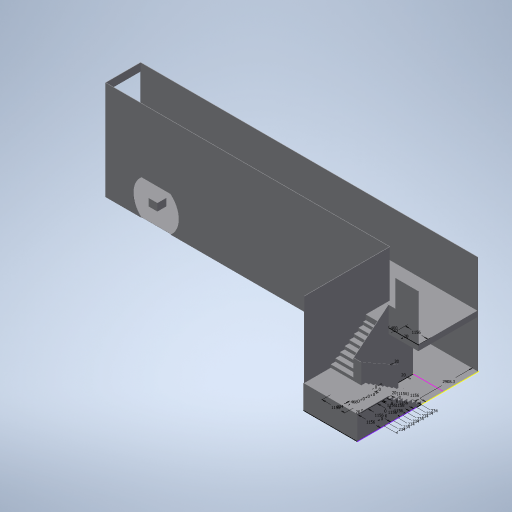
# Autodesk Inventor part: ATF_Corridors_Drawing
Saved by Autodesk Inventor 2023.1 (Build 271208000, 208)
## iProperties
Created: 2014-01-16
Part Number: ATF_Corridors_Drawing
Material: Generic
Document SubType Name: Modeling
Designer: mcgratta
Density: 1 g/cm^3
Appearance: Default
Author: mcgratta
Autodesk Inventor part; units mm, degrees
ref_plane "YZ Plane" through (0, 0, 0) normal (1, 0, 0) x (0, 1, 0)
ref_plane "XZ Plane" through (0, 0, 0) normal (0, 1, 0) x (-1, 0, 0)
sketch "Sketch1" plane through (0, 0, 0) normal (0, 1, 0) x (-1, 0, 0)
  line L0 (0, 0) -> (14380, 0)
  line L1 (14380, 0) -> (14380, -1790)
  line L2 (14380, -1790) -> (0, -1790)
  line L3 (0, -1790) -> (0, 0)
  line L4 (0, -1790) -> (-2720, -1790)
  line L5 (-2720, -1790) -> (-2720, 4350)
  line L6 (-2720, 4350) -> (0, 4350)
  line L7 (0, 4350) -> (0, -1790)
  dimension "d0" = 1790
  dimension "d2" = 14380
  dimension "d3" = 2720
  dimension "d4" = 6140
  constraints: 16 end point, 4 parallel, 2 horizontal, 2 perpendicular
  measures "d0" distance between parallel lines of L0 L2
  measures "d2" distance between parallel lines of L3 L1
  measures "d3" distance between parallel lines of L5 L7
  measures "d4" distance between parallel lines of L6 L4
extrude "Extrusion1" add sketch "Sketch1" along normal blind 10
sketch "Sketch2" plane through (0, 10, 0) normal (0, 1, 0) x (1, 0, 0)
  line L0 (2720, -4350) -> (2720, 1790) projected
  line L1 (0, -4350) -> (2720, -4350)
  line L2 (2720, -4350) -> (2720, -4330)
  line L3 (2720, -4330) -> (0, -4330)
  line L4 (0, -4330) -> (0, -4350)
  dimension "d7" = 20
  constraints: 8 end point, 2 parallel, 1 horizontal, 1 perpendicular, 1 point on line
  measures "d7" distance between parallel lines of L3 L1
extrude "Extrusion2" [suppressed]
sketch "Sketch3" plane through (0, 10, 0) normal (0, 1, 0) x (1, 0, 0)
  line L0 (2720, 1790) -> (-14380, 1790) projected
  line L1 (2720, -4330) -> (2700, -4330)
  line L2 (2700, -4330) -> (2700, 1790)
  line L3 (2700, 1790) -> (2720, 1790)
  line L4 (2720, 1790) -> (2720, -4330)
  dimension "d11" = 20
  constraints: 8 end point, 2 parallel, 1 horizontal, 1 perpendicular, 1 point on line
  measures "d11" distance between parallel lines of L4 L2
sketch "Sketch4" plane through (0, 10, 0) normal (0, 1, 0) x (1, 0, 0)
  line L0 (-14380, 1790) -> (-14380, 0) projected
  line L1 (2700, 1790) -> (-14380, 1790)
  line L2 (-14380, 1790) -> (-14380, 1770)
  line L3 (-14380, 1770) -> (2700, 1770)
  line L4 (2700, 1770) -> (2700, 1790)
  dimension "d15" = 20
  constraints: 8 end point, 2 parallel, 1 horizontal, 1 perpendicular, 1 point on line
  measures "d15" distance between parallel lines of L3 L1
extrude "Extrusion4" add sketch "Sketch4" along normal blind 5000
sketch "Sketch5" plane through (0, 10, 0) normal (0, 1, 0) x (1, 0, 0)
  line L0 (-14380, 0) -> (0, 0) projected
  line L1 (-14380, 1770) -> (-14360, 1770)
  line L2 (-14360, 1770) -> (-14360, 0)
  line L3 (-14360, 0) -> (-14380, 0)
  line L4 (-14380, 0) -> (-14380, 1770)
  dimension "d19" = 20
  constraints: 8 end point, 2 parallel, 1 horizontal, 1 perpendicular, 1 point on line
  measures "d19" distance between parallel lines of L2 L4
extrude "Extrusion5" add sketch "Sketch5" along normal blind 5000
sketch "Sketch6" plane through (0, 10, 0) normal (0, 1, 0) x (1, 0, 0)
  line L0 (-14360, 0) -> (0, 0)
  line L1 (0, 0) -> (0, 20)
  line L2 (0, 20) -> (-14360, 20)
  line L3 (-14360, 20) -> (-14360, 0)
  dimension "d23" = 20
  constraints: 8 end point, 2 parallel, 1 horizontal, 1 perpendicular
  measures "d23" distance between parallel lines of L0 L2
extrude "Extrusion6" add sketch "Sketch6" along normal blind 5000
sketch "Sketch7" plane through (0, 10, 0) normal (0, 1, 0) x (1, 0, 0)
  line L0 (0, 0) -> (0, -4350) projected
  line L1 (0, -4330) -> (2720, -4330) projected
  line L2 (0, 0) -> (20, 0)
  line L3 (20, 0) -> (20, -4330)
  line L4 (20, -4330) -> (0, -4330)
  line L5 (0, -4330) -> (0, 0)
  point P0 (2700, -4330)
  dimension "d27" = 20
  constraints: 8 end point, 2 parallel, 1 horizontal, 1 perpendicular, 1 point on line
  measures "d27" distance between parallel lines of L3 L5
extrude "Extrusion7" add sketch "Sketch7" along normal blind 5000
ref_plane "Work Plane1" through (2690, 10, 4330) normal (-1, 0, 0) x (0, 0, 1)
sketch "Sketch12" plane through (0, 10, 0) normal (0, 1, 0) x (1, 0, 0)
  line L0 (-14360, 1770) -> (-14360, 20) projected
  line L1 (-14360, 20) -> (0, 20) projected
  line L2 (-12860, 1120) -> (-12410, 1120)
  line L3 (-12410, 1120) -> (-12410, 670)
  line L4 (-12410, 670) -> (-12860, 670)
  line L5 (-12860, 670) -> (-12860, 1120)
  dimension "d115" = 1500
  dimension "d116" = 450
  dimension "d117" = 450
  dimension "d118" = 650
  constraints: 8 end point, 2 parallel, 1 horizontal, 1 perpendicular
  measures "d115" distance between parallel lines of L5 L0
  measures "d116" distance between parallel lines of L4 L2
  measures "d117" distance between parallel lines of L3 L5
  measures "d118" distance between parallel lines of L1 L4
extrude "Extrusion12" add sketch "Sketch12" along normal blind 370
sketch "Sketch13" plane through (-14360, 10, -1770) normal (1, 0, 0) x (0, 0, -1)
  line L0 (-1750, 5000) -> (-1750, 0) projected
  line L1 (0, 0) -> (-1750, 0) projected
  line L2 (0, 5000) -> (0, 0) projected
  line L3 (-1750, 5000) -> (0, 5000) projected
  line L4 (-1750, 2650) -> (0, 2650)
  line L5 (0, 2650) -> (0, 2370)
  line L6 (0, 2370) -> (-1750, 2370)
  line L7 (-1750, 2370) -> (-1750, 2650)
  point P0 (-1770, -10)
  dimension "d121" = 2370
  dimension "d122" = 2350
  constraints: 8 end point, 2 parallel, 2 point on line, 1 horizontal, 1 perpendicular
  measures "d121" distance between parallel lines of L1 L6
  measures "d122" distance between parallel lines of L4 L3
extrude "Extrusion13" add sketch "Sketch13" along normal blind 17040 contours L4 L2 L6 L0
sketch "Sketch14" plane through (0, 2380, -20) normal (0, 0, 1) x (1, 0, 0)
  line L0 (0, 0) -> (0, 280) projected
  line L1 (0, 0) -> (2680, 0) projected
  line L2 (0, 280) -> (2680, 280)
  line L3 (2680, 280) -> (2680, 0)
  line L4 (2680, 0) -> (0, 0)
  line L5 (0, 0) -> (0, 280)
  point P0 (0, -2380)
  constraints: 8 end point, 2 parallel, 1 horizontal, 1 perpendicular
extrude "Extrusion14" add sketch "Sketch14" along normal blind 1239
sketch "Sketch16" plane through (-14360, 2660, -20) normal (0, 1, 0) x (1, 0, 0)
  line L0 (17040, -1239) -> (15884, -1239)
  line L1 (15884, -1239) -> (15884, -1219)
  line L2 (15884, -1219) -> (17040, -1219)
  line L3 (17040, -1219) -> (17040, -1239)
  line L4 (15884, -1239) -> (15484, -1239)
  line L5 (15484, -1239) -> (15484, -1219)
  line L6 (15484, -1219) -> (15884, -1219)
  line L7 (15884, -1219) -> (15884, -1239)
  dimension "d168" = 20
  dimension "d170" = 1156
  dimension "d258" = 20
  dimension "d259" = 400
  constraints: 16 end point, 4 parallel, 2 horizontal, 2 perpendicular
  measures "d168" distance between parallel lines of L2 L0
  measures "d170" distance of L2.end L1.end
  measures "d258" distance between parallel lines of L6 L4
  measures "d259" distance of L5.end L6.end
extrude "Extrusion17" add sketch "Sketch16" along normal blind 2347 contours L0 L1 L2 L3
sketch "Sketch17" plane through (-14380, 0, -1790) normal (-1, 0, 0) x (0, 0, 1)
  line L0 (0, 5010) -> (1790, 5010) projected
  line L1 (20, 2663) -> (1770, 2663)
  line L2 (1770, 2663) -> (1770, 4619)
  line L3 (1770, 4619) -> (20, 4619)
  line L4 (20, 4619) -> (20, 2663)
  line L5 (0, 0) -> (0, 5010) projected
  dimension "d179" = 20
  dimension "d180" = 1750
  dimension "d181" = 391
  dimension "d182" = 1956
  constraints: 8 end point, 2 parallel, 1 horizontal, 1 perpendicular
  measures "d179" distance between parallel lines of L5 L4
  measures "d180" distance between parallel lines of L2 L4
  measures "d181" distance between parallel lines of L3 L0
  measures "d182" distance between parallel lines of L1 L3
extrude "Extrusion18" cut sketch "Sketch17" along normal mid plane 50
sketch "Sketch18" plane through (-14380, 0, 0) normal (0, 0, 1) x (1, 0, 0)
  line L0 (0, 0) -> (14380, 0) projected
  arc A0 (3305.7392, 0) -> (1827.2099, 0) centre (2566.4746, 886.2602) ccw
  constraints: 2 point on circle, 2 point on line, 1 centre point
extrude "Extrusion19" cut sketch "Sketch18" along normal mid plane 50
sketch "Sketch19" plane through (0, 10, 0) normal (0, 1, 0) x (1, 0, 0)
  line L0 (2720, -4350) -> (2720, 1790) projected
  line L1 (2720, -1118.3) -> (1564, -1118.3)
  line L2 (1564, -1118.3) -> (1564, -1352.3)
  line L3 (1564, -1352.3) -> (2720, -1352.3)
  line L4 (2720, -1352.3) -> (2720, -1118.3)
  line L5 (2700, 1790) -> (-14380, 1790) projected
  line L6 (2720, -1352.3) -> (1564, -1352.3)
  line L7 (1564, -1352.3) -> (1564, -1586.3)
  line L8 (1564, -1586.3) -> (2720, -1586.3)
  line L9 (2720, -1586.3) -> (2720, -1352.3)
  line L10 (2720, -1586.3) -> (1564, -1586.3)
  line L11 (1564, -1586.3) -> (1564, -1820.3)
  line L12 (1564, -1820.3) -> (2720, -1820.3)
  line L13 (2720, -1820.3) -> (2720, -1586.3)
  line L14 (2720, -1820.3) -> (1564, -1820.3)
  line L15 (1564, -1820.3) -> (1564, -2054.3)
  line L16 (1564, -2054.3) -> (2720, -2054.3)
  line L17 (2720, -2054.3) -> (2720, -1820.3)
  line L18 (2720, -2054.3) -> (1564, -2054.3)
  line L19 (1564, -2054.3) -> (1564, -2288.3)
  line L20 (1564, -2288.3) -> (2720, -2288.3)
  line L21 (2720, -2288.3) -> (2720, -2054.3)
  line L22 (2720, -2288.3) -> (1564, -2288.3)
  line L23 (1564, -2288.3) -> (1564, -2522.3)
  line L24 (1564, -2522.3) -> (2720, -2522.3)
  line L25 (2720, -2522.3) -> (2720, -2288.3)
  line L26 (2720, -2522.3) -> (1564, -2522.3)
  line L27 (1564, -2522.3) -> (1564, -2756.3)
  line L28 (1564, -2756.3) -> (2720, -2756.3)
  line L29 (2720, -2756.3) -> (2720, -2522.3)
  line L30 (2720, -2756.3) -> (1564, -2756.3)
  line L31 (1564, -2756.3) -> (1564, -2990.3)
  line L32 (1564, -2990.3) -> (2720, -2990.3)
  line L33 (2720, -2990.3) -> (2720, -2756.3)
  line L34 (0, 0) -> (0, -4350) projected
  line L35 (2720, -2990.3) -> (0, -2990.3)
  line L36 (0, -2990.3) -> (0, -4350)
  line L37 (0, -4350) -> (2720, -4350)
  line L38 (2720, -4350) -> (2720, -2990.3)
  line L39 (0, -2990.3) -> (1156, -2990.3)
  line L40 (1156, -2990.3) -> (1156, -2756.3)
  line L41 (1156, -2756.3) -> (0, -2756.3)
  line L42 (0, -2756.3) -> (0, -2990.3)
  line L43 (0, -2756.3) -> (1156, -2756.3)
  line L44 (1156, -2756.3) -> (1156, -2522.3)
  line L45 (1156, -2522.3) -> (0, -2522.3)
  line L46 (0, -2522.3) -> (0, -2756.3)
  line L47 (0, -2522.3) -> (1156, -2522.3)
  line L48 (1156, -2522.3) -> (1156, -2288.3)
  line L49 (1156, -2288.3) -> (0, -2288.3)
  line L50 (0, -2288.3) -> (0, -2522.3)
  line L51 (0, -2288.3) -> (1156, -2288.3)
  line L52 (1156, -2288.3) -> (1156, -2054.3)
  line L53 (1156, -2054.3) -> (0, -2054.3)
  line L54 (0, -2054.3) -> (0, -2288.3)
  line L55 (0, -2054.3) -> (1156, -2054.3)
  line L56 (1156, -2054.3) -> (1156, -1820.3)
  line L57 (1156, -1820.3) -> (0, -1820.3)
  line L58 (0, -1820.3) -> (0, -2054.3)
  line L59 (0, -1820.3) -> (1156, -1820.3)
  line L60 (1156, -1820.3) -> (1156, -1586.3)
  line L61 (1156, -1586.3) -> (0, -1586.3)
  line L62 (0, -1586.3) -> (0, -1820.3)
  line L63 (0, -1586.3) -> (1156, -1586.3)
  line L64 (1156, -1586.3) -> (1156, -1352.3)
  line L65 (1156, -1352.3) -> (0, -1352.3)
  line L66 (0, -1352.3) -> (0, -1586.3)
  line L67 (0, -1352.3) -> (1156, -1352.3)
  line L68 (1156, -1352.3) -> (1156, -1118.3)
  line L69 (1156, -1118.3) -> (0, -1118.3)
  line L70 (0, -1118.3) -> (0, -1352.3)
  line L71 (-11062.4346, 20) -> (0, 20) projected
  line L72 (0, 20) -> (1156, 20)
  line L73 (1156, 20) -> (1156, 0)
  line L74 (1156, 0) -> (0, 0)
  line L75 (0, 0) -> (0, 20)
  line L76 (0, 20) -> (2680, 20) projected
  line L77 (1156, -2990.3) -> (1176, -2990.3)
  line L78 (1176, -2990.3) -> (1176, 20)
  line L79 (1176, 20) -> (1156, 20)
  line L80 (1156, 20) -> (1156, -2990.3)
  line L81 (1564, -2990.3) -> (1544, -2990.3)
  line L82 (1544, -2990.3) -> (1544, -1118.3)
  line L83 (1544, -1118.3) -> (1564, -1118.3)
  line L84 (1564, -1118.3) -> (1564, -2990.3)
  line L85 (1544, -2990.3) -> (1176, -2990.3)
  line L86 (1176, -2990.3) -> (1176, -2970.3)
  line L87 (1176, -2970.3) -> (1544, -2970.3)
  line L88 (1544, -2970.3) -> (1544, -2990.3)
  point P0 (0, -2756.3)
  point P1 (0, -2522.3)
  point P2 (0, -2288.3)
  point P3 (0, -2054.3)
  point P4 (0, -1820.3)
  point P5 (0, -1586.3)
  point P6 (0, -1352.3)
  point P7 (0, -1118.3)
  dimension "d183" = 2908.3
  dimension "d184" = 234
  dimension "d185" = 1156
  dimension "d186" = 234
  dimension "d187" = 234
  dimension "d188" = 234
  dimension "d189" = 234
  dimension "d190" = 234
  dimension "d191" = 234
  dimension "d192" = 234
  dimension "d193" = 1156
  dimension "d194" = 0
  dimension "d195" = 0
  dimension "d196" = 0
  dimension "d197" = 0
  dimension "d198" = 0
  dimension "d199" = 0
  dimension "d200" = 0
  dimension "d201" = 1156
  dimension "d202" = 1156
  dimension "d203" = 1156
  dimension "d204" = 1156
  dimension "d205" = 1156
  dimension "d206" = 1156
  dimension "d207" = 1156
  dimension "d208" = 234
  dimension "d209" = 1156
  dimension "d210" = 0
  dimension "d211" = 0
  dimension "d212" = 0
  dimension "d213" = 0
  dimension "d214" = 0
  dimension "d215" = 0
  dimension "d216" = 468
  dimension "d251" = 20
  dimension "d252" = 20
  dimension "d253" = 20
  dimension "d268" = 20
  constraints: 168 end point, 42 parallel, 21 horizontal, 21 perpendicular, 3 point on line
  measures "d183" distance between parallel lines of L5 L1
  measures "d184" distance between parallel lines of L1 L3
  measures "d185" distance between parallel lines of L0 L2
  measures "d186" distance between parallel lines of L6 L8
  measures "d187" distance between parallel lines of L10 L12
  measures "d188" distance between parallel lines of L14 L16
  measures "d189" distance between parallel lines of L18 L20
  measures "d190" distance between parallel lines of L22 L24
  measures "d191" distance between parallel lines of L26 L28
  measures "d192" distance between parallel lines of L30 L32
  measures "d193" distance of L1.start L1.end
  measures "d194" distance between parallel lines of L6 L3
  measures "d195" distance between parallel lines of L10 L8
  measures "d196" distance between parallel lines of L12 L14
  measures "d197" distance between parallel lines of L22 L20
  measures "d198" distance between parallel lines of L16 L18
  measures "d199" distance between parallel lines of L24 L26
  measures "d200" distance between parallel lines of L28 L30
  measures "d201" distance between parallel lines of L0 L7
  measures "d202" distance between parallel lines of L0 L11
  measures "d203" distance between parallel lines of L0 L15
  measures "d204" distance between parallel lines of L0 L19
  measures "d205" distance between parallel lines of L0 L23
  measures "d206" distance between parallel lines of L0 L27
  measures "d207" distance between parallel lines of L0 L31
  measures "d208" distance between parallel lines of L41 L35
  measures "d209" distance between parallel lines of L40 L34
  measures "d210" distance between parallel lines of L47 L45
  measures "d211" distance between parallel lines of L51 L49
  measures "d212" distance between parallel lines of L55 L53
  measures "d213" distance between parallel lines of L59 L57
  measures "d214" distance between parallel lines of L61 L63
  measures "d215" distance between parallel lines of L65 L67
  measures "d216" distance between parallel lines of L47 L35
  measures "d251" distance between parallel lines of L72 L74
  measures "d252" distance between parallel lines of L78 L80
  measures "d253" distance between parallel lines of L2 L82
  measures "d268" distance between parallel lines of L87 L35
extrude "Extrusion20" add sketch "Sketch19" along normal blind 150 contours L1 L0 L3 L2
extrude "Extrusion21" add sketch "Sketch19" along normal blind 300 contours L8 L7 L3 L0
extrude "Extrusion22" add sketch "Sketch19" along normal blind 450 contours L12 L11 L8 L0
extrude "Extrusion23" add sketch "Sketch19" along normal blind 600 contours L16 L15 L12 L0
extrude "Extrusion24" add sketch "Sketch19" along normal blind 750 contours L20 L19 L16 L0
extrude "Extrusion25" add sketch "Sketch19" along normal blind 900 contours L24 L23 L20 L0
extrude "Extrusion26" add sketch "Sketch19" along normal blind 1050 contours L28 L27 L24 L0
extrude "Extrusion27" add sketch "Sketch19" along normal blind 1200 contours L32 L31 L28 L0
extrude "Extrusion28" add sketch "Sketch19" along normal blind 1200 contours L37 L34 L35 L32 L0
extrude "Extrusion29" add sketch "Sketch19" along normal blind 1350 contours L34 L41 L40 L35
extrude "Extrusion30" add sketch "Sketch19" along normal blind 1500 contours L34 L45 L44 L41
extrude "Extrusion31" add sketch "Sketch19" along normal blind 1650 contours L34 L49 L48 L45
extrude "Extrusion32" add sketch "Sketch19" along normal blind 1800 contours L34 L53 L52 L49
extrude "Extrusion33" add sketch "Sketch19" along normal blind 1950 contours L34 L57 L56 L53
extrude "Extrusion34" add sketch "Sketch19" along normal blind 2100 contours L34 L61 L60 L57
extrude "Extrusion35" add sketch "Sketch19" along normal blind 2250 contours L34 L65 L64 L61
extrude "Extrusion36" add sketch "Sketch19" along normal blind 2400 contours L68 L65 L34 L69
extrude "Extrusion37" add sketch "Sketch19" along normal blind 2649 contours L73 L74 L75 L72
extrude "Extrusion38" add sketch "Sketch19" along normal blind 2649 contours L40 L44 L48 L52 L56 L60 L64 L68 L80 L73 L76 L78 L35
extrude "Extrusion39" add sketch "Sketch16" along normal blind 1000 contours L4 L5 L6 L1
sketch "Sketch20" plane through (0, 2659, 0) normal (0, 1, 0) x (1, 0, 0)
  line L0 (1176, -2990.3) -> (1564, -2990.3) projected
  line L1 (1176, -2990.3) -> (1156, -2990.3)
  line L2 (1156, -2990.3) -> (1156, -1199.2515)
  line L3 (1156, -1199.2515) -> (1176, -1199.2515)
  line L4 (1176, -1199.2515) -> (1176, -2990.3)
  point P0 (0, 0)
  dimension "d262" = 20
  constraints: 8 end point, 2 parallel, 1 horizontal, 1 perpendicular
  measures "d262" distance between parallel lines of L4 L2
extrude "Extrusion40" add sketch "Sketch20" along normal blind 1000
sketch "Sketch21" plane through (1176, 10, 2990.3) normal (1, 0, 0) x (0, 0, -1)
  point P0 (2990.3, -10)
sketch "Sketch22" plane through (1176, 10, 2990.3) normal (1, 0, 0) x (0, 0, -1)
  line L0 (0, 1200) -> (0, 3649) projected
  line L1 (1771.3, 2650) -> (1771.3, 3650) projected
  line L2 (0, 2200) -> (1771.3, 3650)
  line L3 (0, 1350) -> (0, 3649) projected
  line L4 (0, 2200) -> (0, 3649)
  line L5 (0, 3649) -> (1771.3, 3649) projected
  line L6 (0, 3649) -> (1771.3, 3649)
  point P0 (2990.3, -10)
  point P1 (1770.0784, 3649)
  dimension "d265" = 1000
  constraints: 6 end point, 1 perpendicular, 1 point on line, 1 vertical
  measures "d265" distance of L0.start L2.start
extrude "Extrusion41" cut sketch "Sketch22" against normal blind 30 contours L0 L5 L2
extrude "Extrusion42" add sketch "Sketch19" along normal blind 2207 contours L35 L78 L87 L82
extrude "Extrusion43" add sketch "Sketch19" along normal blind 2207 contours L35 L82 L83 L2 L7 L11 L15 L19 L23 L27 L31
sketch "Sketch23" plane through (1564, 160, 1118.3) normal (1, 0, 0) x (0, 0, -1)
  line L0 (-1873.0069, 2057) -> (18.8323, 1000)
  line L1 (0, 0) -> (0, 2057) projected
  line L2 (18.8323, 1000) -> (0, 2057)
  line L3 (0, 2057) -> (-1873.0069, 2057)
  point P0 (1118.3, -160)
  point P1 (0, 1010.5219)
  dimension "d273" = 1000
  constraints: 6 end point, 1 perpendicular
  measures "d273" vertical distance of L1.start L0.end
extrude "Extrusion44" cut sketch "Sketch23" against normal blind 21 contours L3 L1 L0
body "Solid1"
